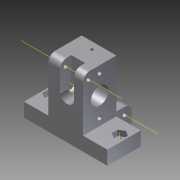
# Autodesk Inventor part: extruder body 175A
Saved by Autodesk Inventor 2012 (Build 160160000, 160)
## iProperties
Created: 2012-01-04
Part Number: extruder body 175A
Material: Default
Document SubType Name: Modeling
Designer: Kennell
Density: 1 g/cm^3
Author: Kennell
Autodesk Inventor part; units mm, degrees
ref_plane "YZ Plane" through (0, 0, 0) normal (1, 0, 0) x (0, 1, 0)
ref_plane "XZ Plane" through (0, 0, 0) normal (0, 1, 0) x (-1, 0, 0)
sketch "Sketch1" plane through (0, 0, 0) normal (0, 0, 1) x (1, 0, 0)
  line L0 (0, 0) -> (60, 0)
  line L1 (60, 0) -> (60, 24)
  line L2 (60, 24) -> (0, 24)
  line L3 (0, 24) -> (0, 0)
  dimension "d0" = 60
  dimension "d1" = 24
  constraints: 8 end point, 2 parallel, 1 horizontal, 1 perpendicular
  measures "d0" distance of L2.end L1.end
  measures "d1" distance of L1.end L0.end
extrude "Extrusion1" add sketch "Sketch1" along normal blind 10
hole "Hole1" at (55, 14, 10) direction (0, 0, -1) diameter 4.5 end through all
hole "Hole2" at (5, 14, 10) direction (0, 0, -1) diameter 4.5 end through all
sketch "Sketch2" plane through (0, 0, 10) normal (0, 0, 1) x (1, 0, 0)
  circle A0 centre (5, 14) radius 2.25 projected
  circle A1 centre (55, 14) radius 2.25 projected
  line L0 (8.75, 16.1651) -> (8.75, 11.8349)
  line L1 (8.75, 11.8349) -> (5, 9.6699)
  line L2 (5, 9.6699) -> (1.25, 11.8349)
  line L3 (1.25, 11.8349) -> (1.25, 16.1651)
  line L4 (1.25, 16.1651) -> (5, 18.3301)
  line L5 (5, 18.3301) -> (8.75, 16.1651)
  line L6 (58.75, 16.1651) -> (58.75, 11.8349)
  line L7 (58.75, 11.8349) -> (55, 9.6699)
  line L8 (55, 9.6699) -> (51.25, 11.8349)
  line L9 (51.25, 11.8349) -> (51.25, 16.1651)
  line L10 (51.25, 16.1651) -> (55, 18.3301)
  line L11 (55, 18.3301) -> (58.75, 16.1651)
  point P0 (1.25, 14)
  dimension "d22" = 7.5
  dimension "d23" = 7.5
  constraints: 24 end point, 2 coincident, 2 vertical, 1 midpoint, 26 other
  measures "d22" distance between parallel lines of L5 L2
  measures "d23" distance between parallel lines of L10 L7
extrude "Extrusion2" cut sketch "Sketch2" against normal blind 4
sketch "Sketch3" plane through (0, 0, 0) normal (0, 0, -1) x (-1, 0, 0)
  line L0 (-60, 24) -> (0, 24)
  point P0 (-30, 19)
  point P1 (-30, 24)
  dimension "d26" = 5
  constraints: 2 end point, 1 midpoint, 1 vertical alignment
  measures "d26" distance of point (-30, 19) point (-30, 24)
hole "Hole3" at (30, 19, 0) direction (0, 0, 1) diameter 16 depth 5.1
hole "Hole4" at (30, 19, 5.1) direction (0, 0, 1) diameter 2 end through all
sketch "Sketch4" plane through (0, 0, 0) normal (0, 0, -1) x (-1, 0, 0)
  arc A0 (-36.245, 24) -> (-23.755, 24) centre (-30, 19) ccw projected
  line L0 (-60, 24) -> (-36.245, 24) projected
  line L1 (-23.755, 24) -> (0, 24) projected
  line L2 (-36.245, 24) -> (-23.755, 24) projected
  line L3 (-23.5, 24) -> (-17.5, 24)
  line L4 (-17.5, 24) -> (-17.5, 35)
  line L5 (-17.5, 35) -> (-23.5, 35)
  line L6 (-23.5, 35) -> (-23.5, 24)
  line L7 (-36.5, 24) -> (-42.5, 24)
  line L8 (-42.5, 24) -> (-42.5, 35)
  line L9 (-42.5, 35) -> (-36.5, 35)
  line L10 (-36.5, 35) -> (-36.5, 24)
  circle A1 centre (-30, 19) radius 1 projected
  dimension "d43" = 6
  dimension "d44" = 11
  dimension "d45" = 6
  dimension "d46" = 11
  dimension "d47" = 25
  dimension "d48" = 12.5
  dimension "d49" = 13
  constraints: 16 end point, 4 parallel, 2 horizontal, 2 perpendicular, 2 point on line
  measures "d43" distance of L5.end L4.end
  measures "d44" distance of L4.end L3.end
  measures "d45" distance of L8.end L9.end
  measures "d46" distance of L7.end L8.end
  measures "d47" distance of L4.end L8.end
  measures "d48" horizontal distance of L3.end A1.centre
  measures "d49" distance between parallel lines of L6 L10
extrude "Extrusion3" add sketch "Sketch4" against normal blind 13 contours L8 L9 L10 L0 | L6 L5 L4 L1
hole "Hole5" at (42.5, 30, 8) direction (-1, 0, 0) diameter 3 end through all
fillet "Fillet1" radius 5 2 edges at (39.5, 35, 13) (20.5, 35, 13)
sketch "Sketch5" plane through (0, 0, 10) normal (0, 0, 1) x (1, 0, 0)
  circle A0 centre (30, 19) radius 1 projected
  line L0 (60, 0) -> (0, 0) projected
  line L1 (17.5, 24) -> (42.5, 24)
  line L2 (42.5, 24) -> (42.5, 0)
  line L3 (42.5, 0) -> (17.5, 0)
  line L4 (17.5, 0) -> (17.5, 24)
  line L5 (42.5, 30) -> (42.5, 24) projected
  constraints: 8 end point, 2 parallel, 1 collinear, 1 horizontal, 1 perpendicular, 1 point on line
extrude "Extrusion4" add sketch "Sketch5" along normal blind 38
hole "Hole6" at (17.5, 12, 29) direction (1, 0, 0) diameter 12.5 end through all
hole "Hole7" at (17.5, 12, 29) direction (1, 0, 0) diameter 23 depth 3 tip angle 118
hole "Hole8" at (17.5, 12, 15) direction (1, 0, 0) diameter 3 end through all
hole "Hole9" at (17.5, 12, 43) direction (1, 0, 0) diameter 3 end through all
sketch "Sketch6" plane through (0, 0, 0) normal (0, -1, 0) x (1, 0, 0)
  line L0 (17.5, 10) -> (17.5, 48) projected
  line L1 (17.5, 10) -> (0, 10) projected
  line L2 (42.5, 35.25) -> (23.6545, 35.25) projected
  line L3 (42.5, 22.75) -> (23.6545, 22.75) projected
  line L4 (20.5, 40.5) -> (20.5, 17.5) projected
  line L5 (23.6545, 22.75) -> (20.5, 17.5) projected
  line L6 (23.6545, 35.25) -> (20.5, 40.5) projected
  line L7 (20.5, 40.5) -> (17.5, 40.5) projected
  line L8 (31, 48) -> (31, 5.1) projected
  line L9 (17.5, 33) -> (20.5, 33)
  line L10 (20.5, 33) -> (20.5, 25)
  line L11 (20.5, 25) -> (17.5, 25)
  line L12 (17.5, 25) -> (17.5, 33)
  point P0 (31, 29)
  dimension "d104" = 8
  dimension "d105" = 15
  dimension "d106" = 3
  dimension "d107" = 19
  constraints: 8 end point, 3 point on line, 2 parallel, 1 horizontal, 1 perpendicular
  measures "d104" distance of L11.end L9.start
  measures "d105" distance of L11.end L0.start
  measures "d106" distance of L10.end L11.end
  measures "d107" distance from line of point (31, 29) L1
hole "Hole10" at (31, 0, 29) direction (0, 1, 0) diameter 10 depth 10 tip angle 118
ref_plane "Work Plane1" through (34.5, 24, 0) normal (1, 0, 0) x (0, 0, -1)
sketch "Sketch7" plane through (34.5, 24, 0) normal (1, 0, 0) x (0, 0, -1)
  circle A0 centre (-29, -12) radius 6.25 projected
  circle A1 centre (-29, -12) radius 11.5 projected
  circle A2 centre (-29, -12) radius 11.5 projected
  circle A3 centre (-29, -12) radius 6.25 projected
  line L0 (-34, -15.75) -> (-34, -24) projected
  line L1 (-24, -15.75) -> (-24, -24) projected
  line L2 (-24, -24) -> (-34, -24) projected
  circle A4 centre (-15, -12) radius 1.5 projected
  circle A5 centre (-43, -12) radius 1.5 projected
  line L3 (-48, -4) -> (-5.1, -4) projected
  line L4 (-48, -6) -> (-5.1, -6) projected
  line L5 (-13, 0) -> (-48, 0) projected
  line L6 (-48, -24) -> (-48, 0) projected
  arc A6 (-39.7766, 0) -> (-18.2234, 0) centre (-29, 8) ccw
  line L7 (-18.2234, 0) -> (-39.7766, 0)
  point P0 (0, -24)
  dimension "d116" = 12
  constraints: 2 end point, 2 point on circle, 1 centre point, 1 coincident, 1 collinear, 1 point on line, 1 vertical alignment
  measures "d116" distance from line of point (-29, 8) L3
extrude "Extrusion5" cut sketch "Sketch7" against normal blind 10 contours A6 L5 A1 | A1 A6 L3 | L3 A6 picked at (-29, -2.8333)
sketch "Sketch8" plane through (23.755, 24, 5.1) normal (0, 1, 0) x (1, 0, 0)
  line L0 (10.745, -13.1234) -> (10.745, -34.6766) projected
  line L1 (0.745, -34.6766) -> (0.745, -13.1234) projected
  line L2 (-6.255, -42.9) -> (18.745, -42.9) projected
  line L3 (0.745, -20.9) -> (10.745, -20.9)
  line L4 (10.745, -20.9) -> (10.745, -26.9)
  line L5 (10.745, -26.9) -> (0.745, -26.9)
  line L6 (0.745, -26.9) -> (0.745, -20.9)
  point P0 (-23.755, 5.1)
  dimension "d119" = 6
  dimension "d120" = 16
  constraints: 8 end point, 2 parallel, 2 point on line, 1 horizontal, 1 perpendicular
  measures "d119" distance between parallel lines of L5 L3
  measures "d120" distance between parallel lines of L5 L2
extrude "Extrusion6" cut sketch "Sketch8" against normal blind 10
sketch "Sketch9" plane through (0, 0, 48) normal (0, 0, 1) x (1, 0, 0)
  line L0 (42.5, 0) -> (17.5, 0) projected
  line L1 (36, 5.75) -> (36, 0) projected
  line L2 (26, 5.75) -> (26, 0) projected
  line L3 (36, 0) -> (26, 0)
  line L4 (26, 0) -> (26, 8)
  line L5 (26, 8) -> (36, 8)
  line L6 (36, 8) -> (36, 0)
  point P0 (0, 0)
  dimension "d123" = 10
  dimension "d124" = 8
  constraints: 8 end point, 2 parallel, 1 horizontal, 1 perpendicular
  measures "d123" distance of L4.end L5.end
  measures "d124" distance of L3.end L4.end
extrude "Extrusion7" cut sketch "Sketch9" against normal blind 20
hole "Hole11" at (42.5, 4, 43) direction (-1, 0, 0) diameter 3 end through all
sketch "Sketch11" plane through (42.5, 24, 0) normal (1, 0, 0) x (0, 0, -1)
  circle A0 centre (-8, 6) radius 1.5 projected
  arc A1 (-48, -20) -> (-46, -24) centre (-43, -20) ccw projected
  line L0 (-10, -24) -> (-48, -24) projected
  line L1 (-10, 0) -> (-10, -24) projected
  line L2 (0, 0) -> (-10, 0) projected
  line L3 (0, 11) -> (0, 0) projected
  line L4 (0, 11) -> (-8, 11) projected
  arc A2 (-8, 11) -> (-13, 6) centre (-8, 6) ccw projected
  line L5 (-13, 6) -> (-13, 0) projected
  line L6 (-13, 0) -> (-48, 0) projected
  line L7 (-48, 0) -> (-48, -24) projected
  circle A3 centre (-29, -12) radius 6.25 projected
  circle A4 centre (-15, -12) radius 1.5 projected
  circle A5 centre (-43, -12) radius 1.5 projected
  circle A6 centre (-43, -20) radius 1.5 projected
  point P0 (0, -24)
  dimension "d138" = 21
  dimension "d139" = 5
  dimension "d140" = 4
  measures "d138" horizontal distance of A3.centre A0.centre
  measures "d139" distance of A1.start A1.centre
  measures "d140" distance from line of L0 A1.centre
fillet "Fillet2" radius 5 2 edges at (39.25, 0, 48) (21.75, 0, 48)
body "Solid1"
